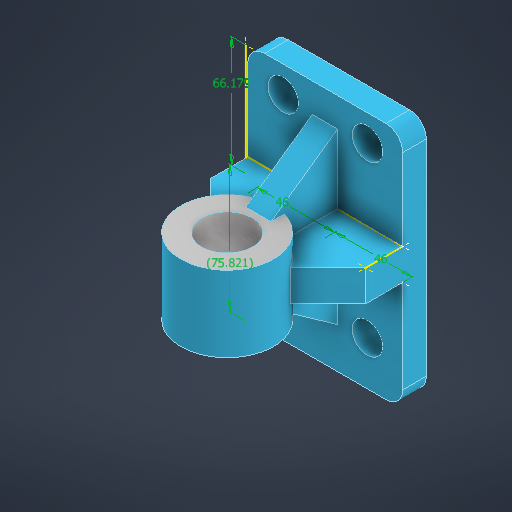
# Autodesk Inventor part: Part6
Saved by Autodesk Inventor 2026.2 (Build 302298000, 298)
## iProperties
Created: 2026-03-25
Part Number: Part6
Material: Nickel-Copper Alloy 400
Document SubType Name: Modeling
Designer: LENOVO
Density: 8.83 g/cm^3
Appearance: Turquoise
Author: LENOVO
Autodesk Inventor part; units mm, degrees
sketch "Sketch1" plane through (0, 0, 0) normal (0, 0, 1) x (1, 0, 0)
  line L0 (-41.267, 50.1755) -> (50.733, 50.1755)
  line L1 (50.733, 50.1755) -> (50.733, -91.8245)
  line L2 (50.733, -91.8245) -> (-41.267, -91.8245)
  line L3 (-41.267, -91.8245) -> (-41.267, 50.1755)
  point P0 (0, 0)
  dimension "d0" = 142
  dimension "d1" = 92
  constraints: 8 end point, 2 parallel, 1 horizontal, 1 perpendicular
  measures "d0" distance of L0.end L1.end
  measures "d1" distance of L1.end L2.end
extrude "Extrusion1" add sketch "Sketch1" along normal blind 14
sketch "Sketch2" plane through (0, 0, 14) normal (0, 0, 1) x (1, 0, 0)
  line L0 (50.733, 50.1755) -> (-41.267, 50.1755) projected
  line L1 (-41.267, -91.8245) -> (50.733, -91.8245) projected
  line L2 (50.733, -91.8245) -> (50.733, 50.1755) projected
  line L3 (50.733, 50.1755) -> (-41.267, 50.1755) projected
  line L4 (-41.267, 50.1755) -> (-41.267, -91.8245) projected
  circle A0 centre (29.733, 34.3976) radius 9
  circle A1 centre (-20.267, 34.3976) radius 9
  circle A2 centre (-20.267, -65.6024) radius 9
  circle A3 centre (29.733, -65.6024) radius 9
  point P0 (0, 0)
  point P1 (-20.267, 50.1755)
  point P2 (29.733, 50.1755)
  point P3 (50.733, 29.1755)
  point P4 (-41.267, 29.1755)
  point P5 (-41.267, 29.1755)
  point P6 (-20.267, 50.1755)
  point P7 (50.733, 29.1755)
  dimension "d5" = 21
  dimension "d6" = 21
  dimension "d7" = 50
  dimension "d8" = 21
  dimension "d9" = 21
  dimension "d13" = 18
  dimension "d14" = 18
  dimension "d15" = 100
  dimension "d16" = 100
  dimension "d17" = 18
  dimension "d18" = 18
  constraints: 9 coincident, 4 centre point, 4 point on line
  measures "d5" distance of point (50.733, 50.176) point (29.733, 50.176)
  measures "d6" distance of point (-20.267, 50.176) L3.end
  measures "d7" distance of point (29.733, 50.176) point (-20.267, 50.176)
  measures "d8" distance of point (50.733, 50.176) point (50.733, 29.176)
  measures "d9" distance of L3.end point (-41.267, 29.176)
  measures "d13" diameter of A1
  measures "d14" diameter of A0
  measures "d15" distance of point (29.733, 34.398) point (29.733, -65.602)
  measures "d16" distance of point (-20.267, 34.398) point (-20.267, -65.602)
  measures "d17" diameter of A3
  measures "d18" diameter of A2
extrude "Extrusion2" cut sketch "Sketch2" against normal through all contours A0 | A1 | A2 | A3
sketch "Sketch3" plane through (0, 0, 14) normal (0, 0, 1) x (1, 0, 0)
  circle A0 centre (-20.267, 34.3976) radius 9 projected
  circle A1 centre (29.733, 34.3976) radius 9 projected
  line L0 (50.733, -91.8245) -> (50.733, 50.1755) projected
  line L1 (-41.267, 50.1755) -> (-41.267, -91.8245) projected
  line L2 (50.733, -8.1024) -> (-41.267, -8.1024)
  line L3 (-41.267, -8.1024) -> (-41.267, -26.6259)
  line L4 (-41.267, -26.6259) -> (50.733, -26.6259)
  line L5 (50.733, -26.6259) -> (50.733, -8.1024)
  point P0 (0, 0)
  point P1 (-20.267, -8.1024)
  point P2 (31.8821, -8.1024)
  point P3 (50.733, -81.8245)
  point P4 (50.733, 40.1755)
  point P5 (-41.267, 40.1755)
  point P6 (-41.267, -81.8245)
  dimension "d22" = 42.5
  dimension "d23" = 42.5
  dimension "d54" = 92
  dimension "d55" = 92
  constraints: 8 end point, 2 coincident, 2 parallel, 2 point on line, 1 horizontal, 1 perpendicular
  measures "d22" distance of A0.centre point (-20.267, -8.102)
  measures "d23" vertical distance of A1.centre point (31.882, -8.102)
  measures "d54" distance of L3.end L4.end
  measures "d55" distance of L2.start L2.end
extrude "Extrusion5" add sketch "Sketch3" along normal blind 58 contours L4 L1 L2 L0
chamfer "Chamfer1" distance 36 angle 45 2 edges at (50.733, -17.3641, 72) (-41.267, -17.3641, 72)
sketch "Sketch10" plane through (-41.267, -8.1024, 14) normal (0, 1, 0) x (1, 0, 0)
  line L0 (92, 0) -> (92, -22) projected
  line L1 (0, 0) -> (92, 0) projected
  point P0 (41.267, 14)
  constraints: 1 coincident
sketch "Sketch11" plane through (-41.267, -26.6259, 14) normal (0, -1, 0) x (1, 0, 0)
  line L0 (92, 0) -> (0, 0) projected
  line L1 (36, 58) -> (56, 58) projected
  point P0 (41.267, -14)
  point P1 (46, 58)
  point P2 (46, 0)
  dimension "d64" = 46
  dimension "d65" = 46
  constraints: 1 coincident, 1 midpoint
  measures "d64" distance of L0.end point (46, 0)
  measures "d65" distance of point (92, 0) point (46, 0)
ref_plane "Work Plane6" through (4.5, 0, 0) normal (1, 0, 0) x (0, 1, 0)
sketch "Sketch12" plane through (4.5, 0, 0) normal (1, 0, 0) x (0, 1, 0)
  line L0 (-8.1024, 14) -> (32.8976, 14)
  line L1 (-8.1024, 14) -> (-8.1024, 72)
  line L2 (-8.1024, 72) -> (32.8976, 14)
  line L3 (-26.6259, 14) -> (-67.6259, 14)
  line L4 (-67.6259, 14) -> (-26.6259, 72)
  line L5 (-26.6259, 72) -> (-26.6259, 14)
  point P0 (0, 0)
  dimension "d67" = 41
  dimension "d68" = 41
  constraints: 12 end point, 2 horizontal, 1 perpendicular
  measures "d67" distance of L0.start L0.end
  measures "d68" distance of L3.start L3.end
extrude "Extrusion6" add sketch "Sketch12" along normal mid plane 15
sketch "Sketch13" plane through (0, 0, 0) normal (0, 1, 0) x (-1, 0, 0)
  point P0 (0, 0)
ref_plane "Work Plane7" through (0, -17.5, 0) normal (0, 1, 0) x (-1, 0, 0)
sketch "Sketch14" plane through (0, -17.5, 0) normal (0, 1, 0) x (-1, 0, 0)
  line L0 (3, 72) -> (-12, 72) projected
  circle A0 centre (-4.5, 72) radius 27.5
  circle A1 centre (-4.5, 72) radius 15
  point P0 (0, 0)
  dimension "d72" = 55
  dimension "d73" = 30
  constraints: 2 centre point, 1 coincident, 1 midpoint
  measures "d72" diameter of A0
  measures "d73" diameter of A1
extrude "Extrusion7" add sketch "Sketch14" along normal mid plane 45
ref_plane "Work Plane8" through (0, 0, 15.25) normal (0, 0, 1) x (1, 0, 0)
sketch "Sketch18" plane through (0, 0, 15.25) normal (0, 0, 1) x (1, 0, 0)
  line L0 (-41.267, 50.1755) -> (-41.267, -91.8245) projected
  point P0 (0, 0)
  point P1 (-41.267, -16.0035)
  dimension "d77" = 66.179
  dimension "d78" = 75.821
  constraints: 1 point on line
  measures "d77" distance of L0.start point (-41.267, -16.004)
  measures "d78" distance of L0.end point (-41.267, -16.004)
sketch "Sketch19" plane through (0, 5, 0) normal (0, 1, 0) x (1, 0, 0)
  circle A0 centre (4.5, -72) radius 15 projected
  point P0 (0, 0)
extrude "Extrusion8" cut sketch "Sketch19" against normal blind 45
fillet "Fillet3" radius 10 4 edges at (50.733, -91.8245, 7) (-41.267, 50.1755, 7) (50.733, 50.1755, 7) (-41.267, -91.8245, 7)
body "Solid1"
